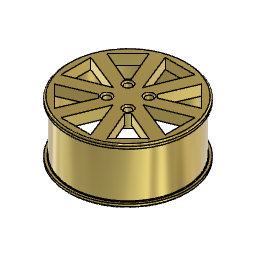
P1 (Autodesk Fusion 360 design; units mm, degrees)
Autodesk Fusion 360 part; units mm, degrees
sketch "Sketch1" plane through (0, 0, 0) normal (0, 1, 0) x (1, 0, 0)
  line L0 (0, 0) -> (190, 0)
  line L1 (0, 0) -> (0, -92.5)
  line L2 (0, -92.5) -> (200, -92.5)
  line L3 (200, -92.5) -> (200, -80)
  line L4 (200, -80) -> (190, -80)
  line L5 (190, -80) -> (190, 0)
  line L6 (190, 80) -> (190, 0)
  line L7 (200, 80) -> (190, 80)
  line L8 (200, 92.5) -> (200, 80)
  line L9 (0, 92.5) -> (200, 92.5)
  line L10 (0, 0) -> (0, 92.5)
  dimension "d3" = 92.5
  dimension "d4" = 200
  dimension "d5" = 12.5
  dimension "d6" = 10
  constraint coincident L0.start L1.start
  constraint horizontal L0
  constraint perpendicular L0 L1
  constraint perpendicular L1 L2
  constraint perpendicular L2 L3
  constraint perpendicular L3 L4
  constraint perpendicular L0 L5
  constraint symmetric L0 L1.start L10.start
  constraint symmetric L0 L1.end L9.start
  constraint symmetric L0 L2.end L8.start
  constraint symmetric L0 L3.end L7.start
  constraint symmetric L0 L4.end L6.start
  constraint symmetric L0 L5.end L6.end
  measures "d3" distance of L0.start L1.end
  measures "d4" distance of L1.end L2.end
  measures "d5" distance of L2.end L3.end
  measures "d6" distance of L3.end L4.end
revolve "Revolve1" add sketch "Sketch1" angle 360 about axis through (0, 0, 0) along (0, 0, -1)
sketch "Sketch2" plane through (0, 0, 92.5) normal (0, 0, 1) x (-1, 0, 0)
  circle A0 centre (0, 0) radius 200
  circle A1 centre (35.3553, -35.3553) radius 11.5
  circle A2 centre (35.3553, 35.3553) radius 11.5
  circle A3 centre (-35.3553, 35.3553) radius 11.5
  circle A4 centre (-35.3553, -35.3553) radius 11.5
  dimension "d11" = 23
  dimension "d13" = 360
  dimension "d14" = 100
  measures "d11" diameter of A1
  measures "d14" distance of A1.centre A3.centre
extrude "Extrude1" cut sketch "Sketch2" against normal through all contours A1 | A2 | A3 | A4
sketch "Sketch3" plane through (0, 0, 92.5) normal (0, 0, 1) x (-1, 0, 0)
  circle A0 centre (35.3553, 35.3553) radius 11.5
  circle A1 centre (-35.3553, 35.3553) radius 11.5
  circle A2 centre (35.3553, -35.3553) radius 11.5
  circle A3 centre (-35.3553, -35.3553) radius 11.5
  circle A4 centre (0, 0) radius 200
  line L0 (0, -175) -> (50, -175)
  line L1 (0, -175) -> (-50, -175)
  line L2 (-50, -175) -> (0, -50)
  line L3 (50, -175) -> (0, -50)
  line L4 (88.3883, -159.099) -> (43.6545, -54.7201)
  line L5 (123.7437, -123.7437) -> (88.3883, -159.099)
  line L6 (123.7437, -123.7437) -> (159.099, -88.3883)
  line L7 (159.099, -88.3883) -> (54.7201, -43.6545)
  line L8 (175, -50) -> (50, 0)
  line L9 (175, 0) -> (175, -50)
  line L10 (175, 0) -> (175, 50)
  line L11 (175, 50) -> (50, 0)
  line L12 (159.099, 88.3883) -> (54.7201, 43.6545)
  line L13 (123.7437, 123.7437) -> (159.099, 88.3883)
  line L14 (123.7437, 123.7437) -> (88.3883, 159.099)
  line L15 (88.3883, 159.099) -> (43.6545, 54.7201)
  line L16 (50, 175) -> (0, 50)
  line L17 (0, 175) -> (50, 175)
  line L18 (0, 175) -> (-50, 175)
  line L19 (-50, 175) -> (0, 50)
  line L20 (-123.7437, 123.7437) -> (-88.3883, 159.099)
  line L21 (-123.7437, 123.7437) -> (-159.099, 88.3883)
  line L22 (-175, 50) -> (-50, 0)
  line L23 (-175, 0) -> (-175, 50)
  line L24 (-175, 0) -> (-175, -50)
  line L25 (-175, -50) -> (-50, 0)
  line L26 (-159.099, -88.3883) -> (-54.7201, -43.6545)
  line L27 (-123.7437, -123.7437) -> (-159.099, -88.3883)
  line L28 (-123.7437, -123.7437) -> (-88.3883, -159.099)
  line L29 (-88.3883, -159.099) -> (-43.6545, -54.7201)
  circle A5 centre (0, 0) radius 70
  line L30 (-88.3883, 159.099) -> (-43.6545, 54.7201)
  line L31 (-159.099, 88.3883) -> (-54.7201, 43.6545)
  dimension "d18" = 50
  dimension "d19" = 125
  dimension "d20" = 50
  dimension "d23" = 140
  constraint coincident A4.centre A5.centre
  constraint coincident A5 L7.end
  constraint coincident A5 L4.end
  constraint coincident A5 L15.end
  constraint coincident A5 L12.end
  constraint coincident A5 L30.end
  constraint coincident A5 L31.end
  constraint coincident A5 L26.end
  constraint coincident A5 L29.end
  measures "d18" distance of A4.centre L2.end
  measures "d19" distance of L2.end L0.start
  measures "d20" distance of L0.start L0.end
  measures "d23" diameter of A5
extrude "Extrude2" cut sketch "Sketch3" against normal through all contours L0 L1 L2 L3 A5 | L2 L3 A5 | L4 L5 L6 L7 A5 | L26 L27 L28 L29 A5 | L8 L9 L10 L11 A5 | L8 L11 A5 | L22 L25 A5 | L22 L23 L24 L25 A5 | L20 L21 A5 L30 L31 | L12 L13 L14 L15 A5 | L16 L19 A5 | L16 L17 L18 L19 A5
sketch "Sketch4" plane through (0, 0, -92.5) normal (0, 0, -1) x (1, 0, 0)
  line L0 (-50, 175) -> (50, 175)
  line L1 (50, 175) -> (0, 50)
  line L2 (0, 50) -> (-50, 175)
  line L3 (50, -175) -> (-50, -175)
  line L4 (-50, -175) -> (0, -50)
  line L5 (0, -50) -> (50, -175)
  line L6 (54.7201, -43.6545) -> (159.099, -88.3883)
  line L7 (159.099, -88.3883) -> (88.3883, -159.099)
  line L8 (88.3883, -159.099) -> (43.6545, -54.7201)
  arc A0 (43.6545, -54.7201) -> (54.7201, -43.6545) centre (0, 0) ccw
  line L9 (-54.7201, 43.6545) -> (-159.099, 88.3883)
  line L10 (-159.099, 88.3883) -> (-88.3883, 159.099)
  line L11 (-88.3883, 159.099) -> (-43.6545, 54.7201)
  arc A1 (-43.6545, 54.7201) -> (-54.7201, 43.6545) centre (0, 0) ccw
  line L12 (43.6545, 54.7201) -> (88.3883, 159.099)
  line L13 (88.3883, 159.099) -> (159.099, 88.3883)
  line L14 (159.099, 88.3883) -> (54.7201, 43.6545)
  arc A2 (54.7201, 43.6545) -> (43.6545, 54.7201) centre (0, 0) ccw
  line L15 (-43.6545, -54.7201) -> (-88.3883, -159.099)
  line L16 (-88.3883, -159.099) -> (-159.099, -88.3883)
  line L17 (-159.099, -88.3883) -> (-54.7201, -43.6545)
  arc A3 (-54.7201, -43.6545) -> (-43.6545, -54.7201) centre (0, 0) ccw
  line L18 (175, 50) -> (175, -50)
  line L19 (175, -50) -> (50, 0)
  line L20 (50, 0) -> (175, 50)
  line L21 (-175, -50) -> (-175, 50)
  line L22 (-175, 50) -> (-50, 0)
  line L23 (-50, 0) -> (-175, -50)
  circle A4 centre (-35.3553, 35.3553) radius 11.5
  circle A5 centre (35.3553, 35.3553) radius 11.5
  circle A6 centre (-35.3553, -35.3553) radius 11.5
  circle A7 centre (35.3553, -35.3553) radius 11.5
  circle A8 centre (0, 0) radius 200
  circle A9 centre (0, 0) radius 70
  circle A10 centre (0, 0) radius 185
  dimension "d25" = 140
  dimension "d26" = 370
  constraint concentric A0 A9
  constraint concentric A9 A10
  measures "d25" diameter of A9
  measures "d26" diameter of A10
extrude "Extrude3" cut sketch "Sketch4" against normal blind 150 contours A10
extrude "Extrude4" cut 1 faces at (-8.9751, 9.1778, -92.5) along direction (0, 0, 1) blind 140
fillet "Fillet1" radius 5 2 edges at (-186.4655, -72.3231, 92.5) (-186.4655, -72.3231, -92.5)
fillet "Fillet2" radius 5 2 edges at (-186.4655, -72.3231, 80) (-186.4655, -72.3231, -80)
chamfer "Chamfer1" distance 5 angle 45 4 edges at (-24.6336, -39.5139, 92.5) (-24.6336, 31.1968, 92.5) (46.0771, 31.1968, 92.5) (46.0771, -39.5139, 92.5)
delete_face "DeleteFace1" 1 faces at (-91.1408, -177.7767, -83.5262)
fillet "Fillet3" radius 2 2 edges at (-177.1422, -68.7069, 80) (-177.1422, -68.7069, -80)
delete_face "DeleteFace2" 1 faces at (-91.1408, -177.7767, 83.5262)
